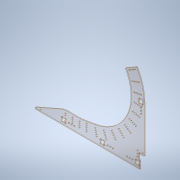
# Autodesk Inventor part: OutsideCLarge_V2
Saved by Autodesk Inventor 2020 (Build 240168000, 168)
## iProperties
Created: 2020-01-19
Part Number: OutsideCLarge_V2
Material: Generic
Document SubType Name: Modeling
Designer: srini
Density: 1 g/cm^3
Appearance: Polycarbonate - Smoked
Author: srini
Autodesk Inventor part; units mm, degrees
ref_plane "YZ Plane" through (0, 0, 0) normal (1, 0, 0) x (0, 1, 0)
ref_plane "XZ Plane" through (0, 0, 0) normal (0, 1, 0) x (-1, 0, 0)
ref_plane "XY Plane" through (0, 0, 0) normal (0, 0, 1) x (1, 0, 0)
sketch "Sketch1" plane through (0, 0, 0) normal (0, 0, 1) x (1, 0, 0)
  line L0 (314.3912, -328.676) -> (351.7292, -328.676)
  line L1 (351.7292, -328.676) -> (351.7292, 0)
  arc A0 (351.7292, 0) -> (297.2819, 203.2) centre (-54.6708, 0) ccw
  line L2 (297.2819, 203.2) -> (214.793, 155.575)
  arc A1 (-1.2995, -306.5385) -> (214.793, 155.575) centre (-54.6708, 0) ccw
  line L3 (-1.2995, -306.5385) -> (-89.9178, -321.9677)
  arc A2 (-111.7019, -323.85) -> (-89.9178, -321.9677) centre (-111.7019, -196.85) ccw
  line L4 (-111.7019, -323.85) -> (-201.2152, -323.85)
  arc A3 (-201.2152, -323.85) -> (-252.0273, -334.4579) centre (-201.2152, -450.85) ccw
  line L5 (-252.0273, -334.4579) -> (-432.5808, -413.2804)
  arc A4 (-432.5808, -413.2804) -> (-430.0402, -425.45) centre (-430.0402, -419.1) ccw
  line L6 (-430.0402, -425.45) -> (314.3912, -425.45)
  line L7 (314.3912, -425.45) -> (314.3912, -328.676)
  line L8 (34.2292, -406.4) -> (34.2292, -381)
  line L9 (34.2292, -381) -> (59.6292, -381)
  line L10 (59.6292, -381) -> (59.6292, -406.4)
  line L11 (59.6292, -406.4) -> (34.2292, -406.4)
  line L12 (313.6292, -406.4) -> (288.2292, -406.4)
  line L13 (288.2292, -406.4) -> (288.2292, -381)
  line L14 (288.2292, -381) -> (313.6292, -381)
  line L15 (313.6292, -381) -> (313.6292, -406.4)
  line L16 (339.0292, -12.7) -> (313.6292, -12.7)
  line L17 (313.6292, -12.7) -> (313.6292, 12.7)
  line L18 (313.6292, 12.7) -> (339.0292, 12.7)
  line L19 (339.0292, 12.7) -> (339.0292, -12.7)
  line L20 (-245.1708, -381) -> (-219.7708, -381)
  line L21 (-219.7708, -381) -> (-219.7708, -406.4)
  line L22 (-219.7708, -406.4) -> (-245.1708, -406.4)
  line L23 (-245.1708, -406.4) -> (-245.1708, -381)
  circle A5 centre (-156.2708, -393.7) radius 3.3734
  circle A6 centre (262.8292, -393.7) radius 3.3734
  circle A7 centre (123.1292, -393.7) radius 3.3734
  circle A8 centre (85.0292, -393.7) radius 3.3734
  circle A9 centre (326.3292, -76.2) radius 3.3734
  circle A10 centre (300.9292, -355.6) radius 3.3734
  circle A11 centre (224.7292, -393.7) radius 3.3734
  circle A12 centre (-175.3208, -393.7) radius 3.3734
  circle A13 centre (243.7792, -393.7) radius 3.3734
  circle A14 centre (300.9292, -317.5) radius 3.3734
  circle A15 centre (326.3292, -57.15) radius 3.3734
  circle A16 centre (104.0792, -393.7) radius 3.3734
  circle A17 centre (300.9292, -336.55) radius 3.3734
  circle A18 centre (326.3292, -38.1) radius 3.3734
  circle A19 centre (-194.3708, -393.7) radius 3.3734
  point P0 (0, 0)
  point P1 (351.7292, 0)
  point P2 (297.2819, 203.2)
  point P3 (214.793, 155.575)
  point P4 (-1.2995, -306.5385)
  point P5 (-89.9178, -321.9677)
  constraints: 48 end point, 20 centre point, 10 point on circle
extrude "Extrusion1" add sketch "Sketch1" along normal blind 6.35
sketch "Sketch2" plane through (0, 0, 6.35) normal (0, 0, 1) x (1, 0, 0)
  line L0 (314.3912, -425.45) -> (314.3912, -328.676) projected
  line L1 (314.3912, -368.3) -> (320.7412, -368.3)
  line L2 (320.7412, -368.3) -> (320.7412, -425.45)
  line L3 (320.7412, -425.45) -> (314.3912, -425.45)
  line L4 (314.3912, -425.45) -> (314.3912, -368.3)
  line L5 (-430.0402, -425.45) -> (314.3912, -425.45) projected
  line L6 (288.2292, -381) -> (313.6292, -381) projected
  point P0 (0, 0)
  dimension "d2" = 6.35
  dimension "d3" = 12.7
  constraints: 8 end point, 2 parallel, 1 collinear, 1 horizontal, 1 perpendicular, 1 point on line
  measures "d2" distance of L1.start L1.end
  measures "d3" distance between parallel lines of L6 L1
extrude "Extrusion2" add sketch "Sketch2" against normal blind 6.35
sketch "Sketch3" plane through (0, 0, 6.35) normal (0, 0, 1) x (1, 0, 0)
  line L0 (313.6292, -12.7) -> (313.6292, 12.7) projected
  circle A0 centre (313.6292, 12.7) radius 3.81
  circle A1 centre (313.6292, -12.7) radius 3.81
  line L1 (339.0292, 12.7) -> (339.0292, -12.7) projected
  circle A2 centre (339.0292, -12.7) radius 3.81
  line L2 (313.6292, 12.7) -> (339.0292, 12.7) projected
  circle A3 centre (339.0292, 12.7) radius 3.81
  line L3 (-245.1708, -381) -> (-219.7708, -381) projected
  circle A4 centre (-245.1708, -381) radius 3.81
  line L4 (-219.7708, -406.4) -> (-245.1708, -406.4) projected
  circle A5 centre (-245.1708, -406.4) radius 3.81
  circle A6 centre (-219.7708, -406.4) radius 3.81
  circle A7 centre (-219.7708, -381) radius 3.81
  line L5 (34.2292, -406.4) -> (34.2292, -381) projected
  circle A8 centre (34.2292, -381) radius 3.81
  circle A9 centre (34.2292, -406.4) radius 3.81
  line L6 (59.6292, -381) -> (59.6292, -406.4) projected
  circle A10 centre (59.6292, -406.4) radius 3.81
  circle A11 centre (59.6292, -381) radius 3.81
  line L7 (288.2292, -406.4) -> (288.2292, -381) projected
  circle A12 centre (288.2292, -381) radius 3.81
  circle A13 centre (288.2292, -406.4) radius 3.81
  line L8 (313.6292, -406.4) -> (288.2292, -406.4) projected
  circle A14 centre (313.6292, -406.4) radius 3.81
  line L9 (313.6292, -381) -> (313.6292, -406.4) projected
  circle A15 centre (313.6292, -381) radius 3.81
  line L10 (314.3912, -328.676) -> (351.7292, -328.676) projected
  circle A16 centre (314.3912, -328.676) radius 3.81
  point P0 (0, 0)
  dimension "d6" = 7.62
  constraints: 17 centre point, 16 equal radius, 6 coincident
  measures "d6" diameter of A1
extrude "Extrusion3" cut sketch "Sketch3" against normal through all
fillet "Fillet1" radius 3.175 40 edges at (-241.3608, -381, 3.175) (-245.1708, -384.81, 3.175) (-245.1708, -402.59, 3.175) (-241.3608, -406.4, 3.175) (-223.5808, -406.4, 3.175) (-223.5808, -381, 3.175) (-219.7708, -384.81, 3.175) (-219.7708, -402.59, 3.175) (38.0392, -381, 3.175) (34.2292, -384.81, 3.175) (34.2292, -402.59, 3.175) (38.0392, -406.4, 3.175) (55.8192, -406.4, 3.175) (59.6292, -402.59, 3.175) (55.8192, -381, 3.175) (59.6292, -384.81, 3.175) (292.0392, -381, 3.175) (288.2292, -384.81, 3.175) (288.2292, -402.59, 3.175) (292.0392, -406.4, 3.175) (309.8192, -406.4, 3.175) (313.6292, -402.59, 3.175) (313.6292, -384.81, 3.175) (309.8192, -381, 3.175) (317.4392, 12.7, 3.175) (313.6292, 8.89, 3.175) (313.6292, -8.89, 3.175) (317.4392, -12.7, 3.175) (335.2192, -12.7, 3.175) (339.0292, -8.89, 3.175) (339.0292, 8.89, 3.175) (335.2192, 12.7, 3.175) (320.7412, -368.3, 3.175) (320.7412, -425.45, 3.175) (351.7292, -328.676, 3.175) (214.793, 155.575, 3.175) (297.2819, 203.2, 3.175) (314.3912, -332.486, 3.175) (318.2012, -328.676, 3.175) (314.3912, -368.3, 3.175)
sketch "Sketch4" plane through (0, 0, 6.35) normal (0, 0, 1) x (1, 0, 0)
  circle A0 centre (240.3781, 155.6818) radius 2.5797
  circle A1 centre (284.3722, 181.0818) radius 2.5797
  line L0 (240.3781, 155.6818) -> (284.3722, 181.0818) construction
  line L1 (294.5215, 201.6062) -> (217.5288, 157.1545) projected
  line L2 (262.3751, 168.3818) -> (256.0251, 179.3804) construction
  circle A2 centre (339.0292, -315.976) radius 2.5797
  line L3 (320.6129, -328.676) -> (348.5542, -328.676) projected
  line L4 (351.7292, -325.501) -> (351.7292, 0) projected
  circle A3 centre (-399.6235, -412.75) radius 2.5797
  line L5 (-430.0402, -425.45) -> (317.5662, -425.45) projected
  line L6 (-252.0273, -334.4579) -> (-432.5808, -413.2804) projected
  arc A4 (-1.2995, -306.5385) -> (216.3507, 152.8452) centre (-54.6708, 0) ccw projected
  circle A5 centre (262.3751, 168.3818) radius 2.5797
  circle A6 centre (251.3766, 162.0318) radius 2.5797
  circle A7 centre (273.3736, 174.7318) radius 2.5797
  circle A8 centre (312.5152, 113.6452) radius 2.5797
  circle A9 centre (288.5122, 105.3376) radius 2.5797
  line L7 (264.5091, 97.0301) -> (312.5152, 113.6452) construction
  circle A10 centre (300.5137, 109.4914) radius 2.5797
  circle A11 centre (276.5107, 101.1839) radius 2.5797
  circle A12 centre (264.5091, 97.0301) radius 2.5797
  circle A13 centre (327.3871, 42.101) radius 2.5797
  circle A14 centre (302.2457, 38.4862) radius 2.5797
  line L8 (277.1042, 34.8714) -> (327.3871, 42.101) construction
  circle A15 centre (314.8164, 40.2936) radius 2.5797
  circle A16 centre (289.6749, 36.6788) radius 2.5797
  circle A17 centre (277.1042, 34.8714) radius 2.5797
  circle A18 centre (328.4505, -30.9647) radius 2.5797
  circle A19 centre (303.0793, -29.7561) radius 2.5797
  line L9 (277.7081, -28.5476) -> (328.4505, -30.9647) construction
  circle A20 centre (315.7649, -30.3604) radius 2.5797
  circle A21 centre (290.3937, -29.1518) radius 2.5797
  circle A22 centre (277.7081, -28.5476) radius 2.5797
  circle A23 centre (315.6669, -102.9113) radius 2.5797
  circle A24 centre (290.9829, -96.9231) radius 2.5797
  line L10 (266.2989, -90.9348) -> (315.6669, -102.9113) construction
  circle A25 centre (303.3249, -99.9172) radius 2.5797
  circle A26 centre (278.6409, -93.9289) radius 2.5797
  circle A27 centre (266.2989, -90.9348) radius 2.5797
  circle A28 centre (289.4983, -171.1385) radius 2.5797
  circle A29 centre (266.3937, -160.5869) radius 2.5797
  line L11 (243.289, -150.0354) -> (289.4983, -171.1385) construction
  circle A30 centre (277.946, -165.8627) radius 2.5797
  circle A31 centre (254.8414, -155.3111) radius 2.5797
  circle A32 centre (243.289, -150.0354) radius 2.5797
  circle A33 centre (250.8906, -233.1802) radius 2.5797
  circle A34 centre (230.2004, -218.4468) radius 2.5797
  line L12 (209.5101, -203.7133) -> (250.8906, -233.1802) construction
  circle A35 centre (240.5455, -225.8135) radius 2.5797
  circle A36 centre (219.8552, -211.08) radius 2.5797
  circle A37 centre (209.5101, -203.7133) radius 2.5797
  circle A38 centre (201.2391, -286.7942) radius 2.5797
  circle A39 centre (183.711, -268.4114) radius 2.5797
  line L13 (166.183, -250.0285) -> (201.2391, -286.7942) construction
  circle A40 centre (192.475, -277.6028) radius 2.5797
  circle A41 centre (174.947, -259.2199) radius 2.5797
  circle A42 centre (166.183, -250.0285) radius 2.5797
  circle A43 centre (142.3383, -330.0427) radius 2.5797
  circle A44 centre (128.606, -308.6749) radius 2.5797
  line L14 (114.8737, -287.307) -> (142.3383, -330.0427) construction
  circle A45 centre (135.4721, -319.3588) radius 2.5797
  circle A46 centre (121.7399, -297.991) radius 2.5797
  circle A47 centre (114.8737, -287.307) radius 2.5797
  circle A48 centre (76.3171, -361.3626) radius 2.5797
  circle A49 centre (66.8768, -337.7821) radius 2.5797
  line L15 (57.4366, -314.2015) -> (76.3171, -361.3626) construction
  circle A50 centre (71.597, -349.5723) radius 2.5797
  circle A51 centre (62.1567, -325.9918) radius 2.5797
  circle A52 centre (57.4366, -314.2015) radius 2.5797
  circle A53 centre (5.5616, -379.6219) radius 2.5797
  circle A54 centre (0.7546, -354.6809) radius 2.5797
  line L16 (-4.0523, -329.74) -> (5.5616, -379.6219) construction
  circle A55 centre (3.1581, -367.1514) radius 2.5797
  circle A56 centre (-1.6489, -342.2105) radius 2.5797
  circle A57 centre (-4.0523, -329.74) radius 2.5797
  circle A58 centre (-67.3708, -384.1607) radius 2.5797
  circle A59 centre (-67.3708, -358.7607) radius 2.5797
  line L17 (-67.3708, -333.3607) -> (-67.3708, -384.1607) construction
  circle A60 centre (-67.3708, -371.4607) radius 2.5797
  circle A61 centre (-67.3708, -346.0607) radius 2.5797
  circle A62 centre (-67.3708, -333.3607) radius 2.5797
  circle A63 centre (-118.1708, -371.4607) radius 2.5797
  circle A64 centre (-118.1708, -384.1607) radius 2.5797
  circle A65 centre (-118.1708, -358.7607) radius 2.5797
  circle A66 centre (-118.1708, -346.0607) radius 2.5797
  circle A67 centre (-168.9708, -371.4607) radius 2.5797
  circle A68 centre (-168.9708, -384.1607) radius 2.5797
  circle A69 centre (-168.9708, -358.7607) radius 2.5797
  circle A70 centre (-168.9708, -346.0607) radius 2.5797
  circle A71 centre (-219.7708, -371.4607) radius 2.5797
  circle A72 centre (-219.7708, -384.1607) radius 2.5797
  circle A73 centre (-219.7708, -358.7607) radius 2.5797
  circle A74 centre (-219.7708, -346.0607) radius 2.5797
  point P0 (0, 0)
  dimension "d10" = 5.1594
  dimension "d11" = 12.7
  dimension "d12" = 50.8
  dimension "d13" = 12.7
  dimension "d14" = 12.7
  dimension "d15" = 12.7
  dimension "d16" = 12.7
  dimension "d17" = 333.6026
  dimension "d18" = 12.7
  dimension "d19" = 12.7
  dimension "d22" = 120
  dimension "d26" = 50.8
  constraints: 74 centre point, 26 end point, 24 point on line, 15 coincident, 6 equal radius, 2 midpoint, 1 horizontal, 1 parallel, 1 perpendicular, 160 other
  measures "d10" diameter of A0
  measures "d11" distance of L2.start L2.end
  measures "d12" distance of L0.start L0.end
  measures "d13" distance from line of A2.centre L3
  measures "d14" distance from line of A2.centre L4
  measures "d15" distance from line of A3.centre L5
  measures "d16" distance from line of A3.centre L6
  measures "d17" distance of L0.start A4.centre
  measures "d18" distance of L0.start A6.centre
  measures "d19" distance of A5.centre A7.centre
  measures "d26" distance of point (-67.371, -358.761) point (-118.171, -358.761)
extrude "Extrusion4" cut sketch "Sketch4" against normal blind 25.4 contours A0 | A1 | A2 | A3 | A5 | A6 | A7 | A8 | A9 | A10 | A11 | A12 | A13 | A14 | A15 | A16 | A17 | A18 | A19 | A20 | A21 | A22 | A23 | A24 | A25 | A26 | A27 | A28 | A29 | A30 | A31 | A32 | A33 | A34 | A35 | A36 | A37 | A38 | A39 | A40 | A41 | A42 | A43 | A44 | A45 | A46 | A47 | A48 | A49 | A50 | A51 | A52 | A53 | A54 | A55 | A56 | A57 | A58 | A59 | A60 | A61 | A62 | A63 | A64 | A65 | A66 | A67 | A68 | A69 | A70 | A73 | A74
body "Solid1"
